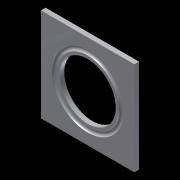
# Autodesk Inventor part: Upper Plate
Saved by Autodesk Inventor 2014 SP1 (Build 180222100, 222)
## iProperties
Created: 2014-04-13
Part Number: Upper Plate
Material: Aluminum 6061
Document SubType Name: Modeling
Designer: Rauhul Varma
Density: 2.71 g/cm^3
Appearance: Aluminum - Flat
Mass: 190.287 g
Surface Area: 285.359 cm^2
Volume: 70.2166 cm^3
Author: Rauhul Varma
Autodesk Inventor part; units mm, degrees
ref_plane "YZ Plane" through (0, 0, 0) normal (1, 0, 0) x (0, 1, 0)
ref_plane "XZ Plane" through (0, 0, 0) normal (0, 1, 0) x (-1, 0, 0)
ref_plane "XY Plane" through (0, 0, 0) normal (0, 0, 1) x (1, 0, 0)
sketch "Sketch1" plane through (0, 0, 0) normal (0, 0, 1) x (1, 0, 0)
  circle A0 centre (0, 0) radius 48.5902 construction
  circle A1 centre (0, 0) radius 42.1132 construction
  circle A2 centre (0, 0) radius 54.61 construction
  circle A3 centre (0, 0) radius 51.7652 construction
  line L0 (0, 0) -> (0, 45.3517) construction
  circle A4 centre (0, 0) radius 38.1
  line L1 (-63.5, -63.5) -> (63.5, -63.5)
  line L2 (63.5, -63.5) -> (63.5, 63.5)
  line L3 (63.5, 63.5) -> (-63.5, 63.5)
  line L4 (-63.5, 63.5) -> (-63.5, -63.5)
  line L5 (-63.5, -63.5) -> (63.5, 63.5) construction
  line L6 (63.5, -63.5) -> (-63.5, 63.5) construction
  dimension "d0" = 97.1804
  dimension "d1" = 84.2264
  dimension "d2" = 109.22
  dimension "d3" = 103.5304
  dimension "d15" = 45.3517
  dimension "d27" = 76.2
  dimension "d28" = 127
  dimension "d29" = 127
  constraints: 14 end point, 5 centre point, 5 coincident, 2 midpoint, 2 parallel, 1 horizontal, 1 perpendicular, 1 vertical
  measures "d0" diameter of A0
  measures "d1" diameter of A1
  measures "d2" diameter of A2
  measures "d3" diameter of A3
  measures "d15" distance of L0.start L0.end
  measures "d27" diameter of A4
  measures "d28" distance of L3.end L2.end
  measures "d29" distance of L2.end L1.end
sketch "Sketch2" plane through (0, 0, 0) normal (1, 0, 0) x (0, 1, 0)
  line L0 (0, 0) -> (45.3517, 0) construction
  line L1 (45.3517, 0) -> (45.3517, 0.7937) construction
  circle A0 centre (45.3517, 0.7937) radius 3.2385
  line L2 (0, 0) -> (0, 25.4) construction
  dimension "d16" = 6.477
  dimension "d17" = 0.7937
  dimension "d18" = 25.4
  constraints: 4 end point, 1 centre point, 1 coincident, 1 parallel, 1 perpendicular
  measures "d16" diameter of A0
  measures "d17" distance of L0.end L1.end
  measures "d18" distance of L0.start L2.end
extrude "Extrusion2" add sketch "Sketch1" against normal blind 6.35
revolve "Revolution2" cut sketch "Sketch2" angle 360 about axis through (0, 0, 0) along (0, 0, 1)
equation "\"d15\" = 0.25 * d1 + 0.25 * d0"
body "Solid2"
